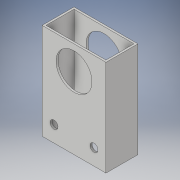
# Autodesk Inventor part: 1x2 hexshaft mount
Saved by Autodesk Inventor 2018 (Build 220112000, 112)
## iProperties
Created: 2020-01-27
Part Number: 1x2 hexshaft mount
Material: Generic
Document SubType Name: Modeling
Designer: Burni
Density: 1 g/cm^3
Appearance: Default
Author: Burni
Autodesk Inventor part; units mm, degrees
ref_plane "YZ Plane" through (0, 0, 0) normal (1, 0, 0) x (0, 1, 0)
ref_plane "XZ Plane" through (0, 0, 0) normal (0, 1, 0) x (-1, 0, 0)
ref_plane "XY Plane" through (0, 0, 0) normal (0, 0, 1) x (1, 0, 0)
sketch "Sketch1" plane through (0, 0, 0) normal (0, 1, 0) x (-1, 0, 0)
  line L0 (-25.4, -12.7) -> (25.4, -12.7)
  line L1 (25.4, -12.7) -> (25.4, 12.7)
  line L2 (25.4, 12.7) -> (-25.4, 12.7)
  line L3 (-25.4, 12.7) -> (-25.4, -12.7)
  line L4 (-25.4, -12.7) -> (25.4, 12.7) construction
  line L5 (25.4, -12.7) -> (-25.4, 12.7) construction
  line L6 (-23.8125, -11.9062) -> (23.8125, 11.9062) construction
  line L7 (23.8125, -11.9062) -> (-23.8125, 11.9062) construction
  line L8 (23.8125, 11.1125) -> (-23.8125, 11.1125)
  line L9 (-23.8125, 11.1125) -> (-23.8125, -11.1125)
  line L10 (-23.8125, -11.1125) -> (23.8125, -11.1125)
  line L11 (23.8125, -11.1125) -> (23.8125, 11.1125)
  point P0 (0, 0)
  dimension "d1" = 25.4
  dimension "d4" = 50.8
  dimension "d7" = 1.5875
  dimension "d8" = 1.5875
  dimension "d9" = 1.5875
  dimension "d10" = 1.5875
  constraints: 24 end point, 4 midpoint, 4 parallel, 2 horizontal, 2 perpendicular, 1 point on line
  measures "d1" distance of L0.end L1.end
  measures "d4" distance of L0.start L0.end
  measures "d7" distance between parallel lines of L1 L11
  measures "d8" distance between parallel lines of L2 L8
  measures "d9" distance between parallel lines of L3 L9
  measures "d10" distance between parallel lines of L10 L0
extrude "Extrusion2" add sketch "Sketch1" along normal blind 76.2
sketch "Sketch2" plane through (-25.4, 0, 12.7) normal (0, 0, 1) x (1, 0, 0)
  circle A0 centre (25.4, 57.15) radius 14.2875
  circle A1 centre (9.525, 12.7) radius 3.175
  circle A2 centre (41.275, 12.7) radius 3.175
  line L0 (0, 0) -> (0, 76.2) projected
  line L1 (0, 0) -> (50.8, 0) projected
  line L2 (0, 76.2) -> (50.8, 76.2) projected
  point P0 (25.4, 0)
  dimension "d13" = 28.575
  dimension "d14" = 31.75
  dimension "d15" = 9.525
  dimension "d16" = 12.7
  dimension "d17" = 12.7
  dimension "d18" = 19.05
  dimension "d19" = 6.35
  dimension "d20" = 6.35
  constraints: 3 centre point
  measures "d13" diameter of A0
  measures "d14" distance of A1.centre A2.centre
  measures "d15" distance from line of L0 A1.centre
  measures "d16" distance from line of L1 A1.centre
  measures "d17" distance from line of L1 A2.centre
  measures "d18" distance from line of L2 A0.centre
  measures "d19" diameter of A1
  measures "d20" diameter of A2
extrude "Extrusion3" cut sketch "Sketch2" against normal blind 76.2
equation "\"d8\" = d7"
equation "\"d9\" = d7"
equation "\"d10\" = d7"
body "Solid2"
